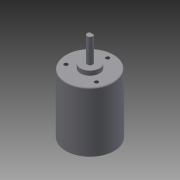
# Autodesk Inventor part: Nidec_DMN37
Saved by Autodesk Inventor 2016 (Build 200138000, 138)
## iProperties
Created: 2016-01-21
Part Number: Nidec_DMN37
Material: Générique
Document SubType Name: Modeling
Designer: sd
Density: 3.17215 g/cm^3
Appearance: Par défaut
Mass: 180 g
Surface Area: 87.8197 cm^2
Volume: 56.7439 cm^3
Author: sd
Autodesk Inventor part; units mm, degrees
ref_plane "YZ Plane" through (0, 0, 0) normal (1, 0, 0) x (0, 1, 0)
ref_plane "XZ Plane" through (0, 0, 0) normal (0, 1, 0) x (-1, 0, 0)
ref_plane "XY Plane" through (0, 0, 0) normal (0, 0, 1) x (1, 0, 0)
sketch "Esquisse1" plane through (0, 0, 0) normal (0, 0, 1) x (1, 0, 0)
  circle A0 centre (0, 0) radius 19.2
  dimension "d0" = 38.4
  constraints: 1 centre point, 1 coincident
  measures "d0" diameter of A0
extrude "Extrusion1" add sketch "Esquisse1" against normal blind 47.5
sketch "Esquisse2" plane through (0, 0, 0) normal (0, 0, 1) x (1, 0, 0)
  circle A0 centre (0, 0) radius 19.2 projected
  circle A1 centre (0, 0) radius 7.5
  dimension "d3" = 15
  constraints: 1 centre point, 1 coincident
  measures "d3" diameter of A1
extrude "Extrusion2" add sketch "Esquisse2" along normal blind 3.5 contours A1
sketch "Esquisse3" plane through (0, 0, 3.5) normal (0, 0, 1) x (1, 0, 0)
  circle A0 centre (0, 0) radius 7.5 projected
  circle A1 centre (0, 0) radius 2.25
  dimension "d6" = 4.5
  constraints: 1 centre point, 1 coincident
  measures "d6" diameter of A1
extrude "Extrusion3" add sketch "Esquisse3" along normal blind 19.5 contours A1
sketch "Esquisse4" plane through (0, 0, -47.5) normal (0, 0, -1) x (-1, 0, 0)
  circle A0 centre (0, 0) radius 19.2 projected
  circle A1 centre (0, 0) radius 7.3
  dimension "d9" = 14.6
  constraints: 1 centre point, 1 coincident
  measures "d9" diameter of A1
extrude "Extrusion4" add sketch "Esquisse4" along normal blind 5.7 contours A1
fillet "Congé1" radius 1 1 edges at (7.3, 0, -53.2)
fillet "Congé2" radius 1 1 edges at (-19.2, 0, 0)
sketch "Esquisse6" plane through (0, 0, 23) normal (0, 0, 1) x (1, 0, 0)
  circle A0 centre (0, 0) radius 2.25 projected
  line L0 (-3, 3.5) -> (3, 3.5)
  line L1 (3, 3.5) -> (3, 1.5)
  line L2 (3, 1.5) -> (-3, 1.5)
  line L3 (-3, 1.5) -> (-3, 3.5)
  dimension "d14" = 1.5
  dimension "d15" = 2
  dimension "d16" = 6
  dimension "d17" = 3
  constraints: 8 end point, 2 parallel, 1 horizontal, 1 perpendicular
  measures "d14" distance from line of L2 A0.centre
  measures "d15" distance of L0.end L1.end
  measures "d16" distance of L0.start L0.end
  measures "d17" horizontal distance of A0.centre L1.end
extrude "Extrusion5" cut sketch "Esquisse6" against normal blind 17 contours L2 A0 | A0 L2 L3 L0 L1 picked at (-0.424, 1.6187)
sketch "Esquisse7" plane through (0, 0, 0) normal (0, 0, 1) x (1, 0, 0)
  circle A0 centre (0, 0) radius 7.5 projected
  circle A1 centre (0, 14) radius 1.5
  dimension "d20" = 3
  dimension "d21" = 14
  constraints: 1 centre point
  measures "d20" diameter of A1
  measures "d21" distance of A0.centre A1.centre
extrude "Extrusion6" cut sketch "Esquisse7" against normal blind 4 contours A1
thread "Filetage1" size "M3x0.5" class "6H" standard "ANSI Metric M Profile" full length
pattern_circular "Réseau circulaire1" count 3 over 360 about axis through (0, 0, 0) along (0, 0, -1) of "Extrusion6"
thread "Filetage2" size "M3x0.5" class "6H" standard "ANSI Metric M Profile" full length
thread "Filetage3" size "M3x0.5" class "6H" standard "ANSI Metric M Profile" full length
equation "\"d17\" = 0.5 * d16"
